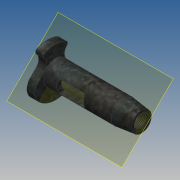
# Autodesk Inventor part: Kurbelwelle_ra8846s
Saved by Autodesk Inventor 2021 (Build 250183000, 183)
## iProperties
Created: 2020-12-18
Part Number: Kurbelwelle_ra8846s
Material: Stahl
Document SubType Name: Modeling
Designer: Sander
Density: 7.85 g/cm^3
Appearance: Platte
Mass: 13.7251 g
Surface Area: 19.4157 cm^2
Volume: 1.74842 cm^3
Author: Sander
Autodesk Inventor part; units mm, degrees
ref_plane "YZ-Ebene" through (0, 0, 0) normal (1, 0, 0) x (0, 1, 0)
ref_plane "XY-Ebene" through (0, 0, 0) normal (0, 0, 1) x (1, 0, 0)
sketch "Skizze1" plane through (0, 0, 0) normal (0, 0, 1) x (1, 0, 0)
  line L0 (-7, 0) -> (42, 0) projected
  line L1 (0, -1.8) -> (0, 10.8) projected
  line L2 (0, 2.8) -> (20, 2.8)
  line L3 (20, 2.8) -> (20, 2.25)
  line L4 (20, 2.25) -> (35, 2.25)
  line L5 (35, 2.25) -> (35, 3.7)
  line L6 (35, 3.7) -> (28.2, 4.5)
  line L7 (28.2, 4.5) -> (3, 4.5)
  line L8 (3, 4.5) -> (3, 9)
  line L9 (3, 9) -> (0, 9)
  line L10 (0, 9) -> (0, 2.8)
  point P0 (0, 0)
  dimension "d0" = 35
  dimension "d1" = 9
  dimension "d2" = 4.5
  dimension "d3" = 2.8
  dimension "d4" = 2.25
  dimension "d5" = 3.7
  dimension "d6" = 3
  dimension "d7" = 6.8
  dimension "d8" = 20
  constraints: 18 end point, 5 perpendicular, 2 point on line, 1 collinear, 1 horizontal, 1 parallel
  measures "d0" horizontal distance of L9.end L5.end
  measures "d1" distance of point (0, 0) L9.end
  measures "d2" distance from line of L0 L6.end
  measures "d3" distance of point (0, 0) L2.start
  measures "d4" distance from line of L0 L4.end
  measures "d5" distance from line of L0 L5.end
  measures "d6" distance of L8.end L9.end
  measures "d7" horizontal distance of L5.end L6.end
  measures "d8" distance of L2.start L2.end
revolve "Umdrehung1" add sketch "Skizze1" angle 360 about axis through (-10, 0, 0) along (1, 0, 0)
chamfer "Fase1" distance 0.5 distance2 0.5 1 edges at (35, -2.25, 0) measured on face at (34.5, -2.25, 0)
ref_plane "Arbeitsebene1" through (15.6, -4.5, 0) normal (0, 1, 0) x (-1, 0, 0)
sketch "Skizze2" plane through (15.6, -4.5, 0) normal (0, 1, 0) x (-1, 0, 0)
  line L0 (15.6, 9) -> (15.6, -9) projected
  line L1 (6.6, 2.4) -> (-1.4, 2.4)
  line L2 (-2.4, 1.4) -> (-2.4, -1.4)
  line L3 (-1.4, -2.4) -> (6.6, -2.4)
  line L4 (7.6, -1.4) -> (7.6, 1.4)
  arc A0 (7.6, 1.4) -> (6.6, 2.4) centre (6.6, 1.4) ccw
  arc A1 (-1.4, 2.4) -> (-2.4, 1.4) centre (-1.4, 1.4) ccw
  arc A2 (-2.4, -1.4) -> (-1.4, -2.4) centre (-1.4, -1.4) ccw
  arc A3 (6.6, -2.4) -> (7.6, -1.4) centre (6.6, -1.4) ccw
  line L5 (12.6, 4.5) -> (12.6, -4.5) projected
  line L6 (-12.6, 4.5) -> (-12.6, -4.5) projected
  line L7 (12.6, 4.5) -> (12.6, -4.5) projected
  line L8 (-4.4, -2.8) -> (15.6, -2.8) projected
  point P0 (15.6, 0)
  point P1 (-2.4, -2.4)
  point P2 (-2.4, 2.4)
  point P3 (7.6, -2.4)
  dimension "d13" = 10
  dimension "d14" = 8
  dimension "d15" = 4.8
  dimension "d16" = 1
  constraints: 8 end point, 8 point on circle, 8 tangent, 6 point on line, 4 centre point, 3 equal radius, 2 parallel, 1 horizontal, 1 perpendicular
  measures "d13" distance of point (7.6, -2.4) point (-2.4, -2.4)
  measures "d14" distance between parallel lines of L4 L0
  measures "d15" distance of point (-2.4, 2.4) point (-2.4, -2.4)
  measures "d16" radius of A0
extrude "Extrusion1" cut sketch "Skizze2" along normal up to next
sketch "Skizze3" plane through (0, 0, 0) normal (-1, 0, 0) x (0, 0, 1)
  circle A0 centre (0, 0) radius 2.8 projected
  circle A1 centre (0, 0) radius 9 projected
  circle A2 centre (-4.1012, 4.1012) radius 1.8
  line L0 (0, -12.6) -> (0, 12.6) projected
  line L1 (0, 0) -> (-4.1012, 4.1012) construction
  dimension "d19" = 3.6
  dimension "d23" = 5.8
  dimension "d24" = 45
  constraints: 2 end point, 1 centre point
  measures "d19" diameter of A2
  measures "d23" distance of L1.end A0.centre
  measures "d24" angle of L0 L1
extrude "Extrusion2" add sketch "Skizze3" along normal blind 4 contours A2
sketch "Skizze4" plane through (0, 0, 0) normal (-1, 0, 0) x (0, 0, 1)
  circle A0 centre (-4.1012, 4.1012) radius 1.8 projected
  circle A1 centre (0, 0) radius 9 projected
  line L0 (0, 0) -> (-4.1012, 4.1012) construction
  arc A2 (0, 6.364) -> (-6.364, 6.364) centre (-3.182, 3.182) ccw
  line L1 (0, 6.364) -> (2.1213, 4.2426)
  arc A3 (2.1213, 4.2426) -> (6.5007, 4.2102) centre (4.3275, 6.4488) ccw
  arc A4 (8.097, 3.9293) -> (6.5007, 4.2102) centre (7.1973, 3.4927) ccw
  dimension "d28" = 9
  dimension "d32" = 4.5
  dimension "d33" = 3.12
  dimension "d34" = 1
  dimension "d36" = 3
  constraints: 8 point on circle, 5 tangent, 4 end point, 3 centre point, 1 parallel
  measures "d28" diameter of A2
  measures "d32" distance between parallel lines of L0 L1
  measures "d33" radius of A3
  measures "d34" radius of A4
  measures "d36" distance of L1.start L1.end
extrude "Extrusion3" cut sketch "Skizze4" against normal through all contours A4 A3 L1 A2 A1 picked at (1.838, 6.3142)
ref_plane "Arbeitsebene2" through (0, 0, 0) normal (0, 0.7071068, 0.7071068) x (1, 0, 0)
mirror "Spiegeln1" about plane through (0, 0, 0) normal (0, 1, 0) of "Extrusion3"
thread "Gewinde1" size "M5x0.5" class "6H" standard "ANSI Metric M Profile" length 15.103
ref_plane "Arbeitsebene3" through (0, 0, 0) normal (0, 0.7071068, -0.7071068) x (1, 0, 0)
